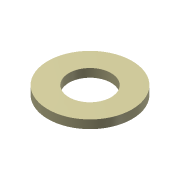
# Autodesk Inventor part: PS20016
Saved by Autodesk Inventor 2014 (Build 180170000, 170)
## iProperties
Category: Need To
Created: 2013-07-25
Part Number: PS20016
Material: Nylon 6/6
Document SubType Name: Modeling
Designer: Edward
Density: 1.13 g/cm^3
Appearance: Nylon 6
Catalog Web Link: http://www.ebay.com/itm/50-Pcs-Nylon-M5-Washer-5mm-x-10mm-x-1mm-thickness-/290925570977?pt=LH_DefaultDomain_0&hash=item43bc83eba1
Description: 5mm x 10mm x 1mm thick,  nylon spacer
Vendor: wongchuham <wongchuham@yahoo.com.hk>
Stock Number: PSM5-01MM
Authority: http://www.ebay.com/itm/50-Pcs-Nylon-M5-Washer-5mm-x-10mm-x-1mm-thickness-/290925570977?pt=LH_DefaultDomain_0&hash=item43bc83eba1
Author: Edward
Subject: Spacers
Comments: Fusion
Title: Large Shim Spacers
Autodesk Inventor part; units mm, degrees
ref_plane "YZ Plane" through (0, 0, 0) normal (1, 0, 0) x (0, 1, 0)
ref_plane "XZ Plane" through (0, 0, 0) normal (0, 1, 0) x (-1, 0, 0)
ref_plane "XY Plane" through (0, 0, 0) normal (0, 0, 1) x (1, 0, 0)
sketch "Sketch1" plane through (0, 0, 0) normal (0, 0, 1) x (1, 0, 0)
  circle A0 centre (0, 0) radius 2.5
  circle A1 centre (0, 0) radius 5
  dimension "d0" = 5
  dimension "d1" = 10
  constraints: 2 centre point, 2 coincident
  measures "d0" diameter of A0
  measures "d1" diameter of A1
extrude "Extrusion1" add sketch "Sketch1" along normal blind 1
body "Solid1"
